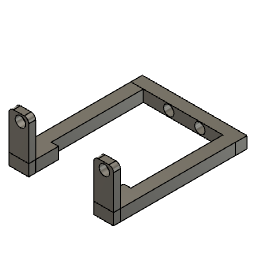
IR holder Line Following (Autodesk Fusion 360 design; units mm, degrees)
Autodesk Fusion 360 part; units mm, degrees
sketch "Sketch1" plane through (0, 0, 0) normal (0, 0, 1) x (1, 0, 0)
  circle A0 centre (35, 52) radius 2.25
  circle A1 centre (71.5, 52) radius 2.25
  line L0 (30, 55) -> (38.6, 55)
  line L1 (38.6, 55) -> (38.6, 33)
  line L2 (38.6, 33) -> (30, 33)
  line L3 (30, 33) -> (30, 55)
  line L4 (66.8505, 55) -> (75.4505, 55)
  line L5 (75.4505, 55) -> (75.4505, 33)
  line L6 (75.4505, 33) -> (66.8505, 33)
  line L7 (66.8505, 33) -> (66.8505, 55)
  line L8 (30, 33) -> (38.6, 33)
  line L9 (38.6, 33) -> (38.6, 38)
  line L10 (38.6, 38) -> (30, 38)
  line L11 (30, 38) -> (30, 33)
  line L12 (66.8505, 33) -> (75.4505, 33)
  line L13 (75.4505, 33) -> (75.4505, 38)
  line L14 (75.4505, 38) -> (66.8505, 38)
  line L15 (66.8505, 38) -> (66.8505, 33)
  dimension "d1" = 4.5
  dimension "d2" = 4.5
  dimension "d3" = 36.5
  dimension "d4" = 22
  dimension "d5" = 3
  dimension "d7" = 22
  dimension "d8" = 8.6
  dimension "d9" = 3
  dimension "d10" = 5
  dimension "d11" = 5
  constraint horizontal L0
  constraint vertical L1
  constraint horizontal L2
  constraint vertical L3
  constraint horizontal L4
  constraint vertical L5
  constraint horizontal L6
  constraint vertical L7
  constraint horizontal L8
  constraint vertical L9
  constraint horizontal L10
  constraint vertical L11
  constraint horizontal L12
  constraint vertical L13
  constraint horizontal L14
  constraint vertical L15
  constraint coincident L5 L13.end
  measures "d1" diameter of A0
  measures "d2" diameter of A1
  measures "d3" distance of A0.centre A1.centre
  measures "d4" distance of L0.start L2.end
  measures "d5" distance of A0.centre L0
  measures "d7" distance of L4.start L6.end
  measures "d8" distance of L0.start L0.end
  measures "d9" distance of A1.centre L4
  measures "d10" distance of L2.end L10.end
  measures "d11" distance of L6.end L14.end
extrude "Extrude1" add sketch "Sketch1" along normal blind 3 contours L0 L1 L3 L10 | L4 L5 L7 L14 makes body 1 at (71.2109, 41.9188, 0) makes body 2 at (34.4773, 41.9188, 0)
extrude "Extrude2" add sketch "Sketch1" against normal blind 50 separate body contours L1 L2 L3 L8 L9 L10 L11 | L5 L6 L7 L12 L13 L14 L15 makes body 3 at (35.7333, 38, -33.3333) makes body 4 at (72.5838, 38, -16.6667)
extrude "Extrude3" add sketch "Sketch1" along normal blind 3 separate body contours L1 L2 L3 L8 L9 L10 L11 | L5 L6 L7 L12 L13 L14 L15 makes body 5 at (32.8667, 36.3333, 0) makes body 6 at (69.7172, 36.3333, 0)
sketch "Sketch2" plane through (30, 0, 0) normal (-1, 0, 0) x (0, 0, 1)
  line L0 (0, 33) -> (0, 38)
  line L1 (0, 38) -> (-50, 38)
  line L2 (-50, 38) -> (-50, 33)
  line L3 (-50, 33) -> (0, 33)
  line L4 (-50, 38) -> (-55, 38)
  line L5 (-55, 38) -> (-55, 33)
  line L6 (-55, 33) -> (-50, 33)
  line L7 (-50, 33) -> (-50, 38)
  dimension "d18" = 5
  constraint horizontal L4
  constraint vertical L5
  constraint horizontal L6
  constraint vertical L7
  constraint coincident L1.end L2.start
  measures "d18" distance of L1.end L2.end
extrude "Extrude4" add sketch "Sketch2" against normal blind 45 separate body contours L2 L4 L5 L6 L7 makes body 7
sketch "Sketch3" plane through (0, 0, -50) normal (0, 0, 1) x (1, 0, 0)
  line L0 (30, 38) -> (30, 33)
  line L1 (30, 33) -> (75, 33)
  line L2 (75, 33) -> (75, 38)
  line L3 (75, 38) -> (30, 38)
  circle A0 centre (46.4611, 35.468) radius 2.25
  circle A1 centre (59.9608, 35.5086) radius 2.25
  dimension "d21" = 4.5
  dimension "d22" = 4.5
  measures "d21" diameter of A0
  measures "d22" diameter of A1
extrude "Extrude5" cut sketch "Sketch3" against normal blind 5 contours A0 | A1 bodies 7
fillet "Fillet1" radius 2 4 edges at (75.4505, 55, 1.5) (66.8505, 55, 1.5) (38.6, 55, 1.5) (30, 55, 1.5) on bodies 1 2
extrude "Extrude6" add 1 faces at (75, 34.6667, -51.6667) along direction (1, 0, 0) blind 0.5 on bodies 7 bodies 7 6 4
sketch "Sketch4" plane through (0, 38, 0) normal (0, 1, 0) x (-1, 0, 0)
  line L0 (-30, -55) -> (-30, -50)
  line L1 (-30, -50) -> (-66.8505, -50)
  line L2 (-66.8505, -50) -> (-66.8505, 0)
  line L3 (-66.8505, 0) -> (-75.4505, 0)
  line L4 (-75.4505, 0) -> (-75.4505, -50)
  line L5 (-75.4505, -50) -> (-75.5, -50)
  line L6 (-75.5, -50) -> (-75.5, -55)
  line L7 (-75.5, -55) -> (-30, -55)
  line L8 (-66.8505, -50) -> (-70, -50)
  line L9 (-70, -50) -> (-70, -10)
  line L10 (-70, -10) -> (-66.8505, -10)
  line L11 (-66.8505, -10) -> (-66.8505, -50)
  line L12 (-38.5651, -50) -> (-35.4151, -50)
  line L13 (-35.4151, -50) -> (-35.4151, -10)
  line L14 (-35.4151, -10) -> (-38.5651, -10)
  line L15 (-38.5651, -10) -> (-38.5651, -50)
  dimension "d28" = 3.15
  dimension "d29" = 40
  constraint horizontal L8
  constraint vertical L9
  constraint horizontal L10
  constraint vertical L11
  constraint coincident L1.end L2.start
  constraint horizontal L12
  constraint vertical L13
  constraint horizontal L14
  constraint vertical L15
  constraint coincident L1 L12.start
  measures "d28" distance of L12.start L12.end
  measures "d29" distance of L12.start L14.end
extrude "Extrude7" cut sketch "Sketch4" against normal blind 10 contours L1 L12 L13 L14 L15 | L2 L8 L9 L10 L11 bodies 3 7
extrude "Extrude8" cut 1 faces at (38.6, 36.3333, -16.6667) along direction (-1, 0, 0) blind 0.05 on bodies 3 bodies 3
